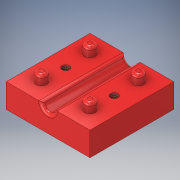
# Autodesk Inventor part: BottomOfSquareSupport
Saved by Autodesk Inventor 2017 SP1 (Build 210196100, 196)
## iProperties
Created: 2015-12-08
Part Number: BottomOfSquareSupport
Material: PC/ABS Plastic
Document SubType Name: Modeling
Designer: steele
Density: 0.357273 g/cm^3
Appearance: Light Red
Author: steele
Autodesk Inventor part; units mm, degrees
ref_plane "YZ Plane" through (0, 0, 0) normal (1, 0, 0) x (0, 1, 0)
ref_plane "XZ Plane" through (0, 0, 0) normal (0, 1, 0) x (-1, 0, 0)
ref_plane "XY Plane" through (0, 0, 0) normal (0, 0, 1) x (1, 0, 0)
sketch "Sketch1" plane through (0, 0, 0) normal (0, 1, 0) x (-1, 0, 0)
  line L0 (-22.225, 22.225) -> (-22.225, -22.225)
  line L1 (-22.225, -22.225) -> (22.225, -22.225)
  line L2 (22.225, -22.225) -> (22.225, 22.225)
  line L3 (22.225, 22.225) -> (-22.225, 22.225)
  line L4 (-22.225, 22.225) -> (22.225, -22.225) construction
  line L5 (-22.225, -22.225) -> (22.225, 22.225) construction
  point P0 (0, 0)
  dimension "d0" = 44.45
  constraints: 12 end point, 2 midpoint, 2 parallel, 2 perpendicular, 1 vertical
  measures "d0" distance of L0.start L0.end
extrude "Extrusion1" add sketch "Sketch1" along normal blind 12.7
sketch "Sketch2" plane through (-22.225, 0, 22.225) normal (0, 0, 1) x (1, 0, 0)
  line L0 (44.45, 12.7) -> (0, 12.7) projected
  arc A0 (18.7325, 12.7) -> (25.7175, 12.7) centre (22.225, 12.7) ccw
  point P0 (22.225, 0)
  dimension "d3" = 6.985
  constraints: 2 point on circle, 2 point on line, 1 centre point, 1 midpoint
  measures "d3" diameter of A0
extrude "Extrusion2" cut sketch "Sketch2" against normal through all
sketch "Sketch3" plane through (0, 0, 0) normal (0, -1, 0) x (1, 0, 0)
  line L0 (-22.225, -22.225) -> (-22.225, 22.225) projected
  line L1 (22.225, 22.225) -> (22.225, -22.225) projected
  line L2 (-22.225, 22.225) -> (-3.4925, 22.225) projected
  line L3 (3.4925, 22.225) -> (22.225, 22.225) projected
  point P0 (0, 0)
  point P1 (-12.8588, 0)
  point P2 (12.8588, 0)
  dimension "d6" = 9.3663
  dimension "d7" = 9.3663
  dimension "d22" = 22.225
  dimension "d23" = 22.225
  measures "d6" distance from line of L0 point (-12.859, 0)
  measures "d7" distance from line of point (12.859, 0) L1
  measures "d22" distance from line of L2 point (-12.859, 0)
  measures "d23" distance from line of L3 point (12.859, 0)
hole "Hole1" at (-12.8588, 0, 0) at (12.8588, 0, 0) direction (0, 1, 0) diameter 3.9624 end through all thread size "10-32 UNF" class "2B" standard "ANSI Unified Screw Threads"
sketch "Sketch7" plane through (0, 12.7, 0) normal (0, 1, 0) x (1, 0, 0)
  line L0 (-12.8588, -12.8588) -> (12.8588, -12.8588) construction
  line L1 (12.8588, -12.8588) -> (12.8588, 12.8588) construction
  line L2 (12.8588, 12.8588) -> (-12.8588, 12.8588) construction
  line L3 (-12.8588, 12.8588) -> (-12.8588, -12.8588) construction
  line L4 (-12.8588, -12.8588) -> (12.8588, 12.8588) construction
  line L5 (12.8588, -12.8588) -> (-12.8588, 12.8588) construction
  line L6 (-22.225, 22.225) -> (-22.225, -22.225) construction
  line L7 (-22.225, -22.225) -> (-3.4925, -22.225) construction
  circle A0 centre (-12.8588, -12.8588) radius 2.7305
  circle A1 centre (-12.8588, 12.8588) radius 2.7305
  circle A2 centre (12.8588, 12.8588) radius 2.7305
  circle A3 centre (12.8588, -12.8588) radius 2.7305
  point P0 (0, 0)
  dimension "d26" = 9.3663
  dimension "d27" = 9.3663
  dimension "d28" = 5.461
  constraints: 12 end point, 4 centre point, 4 coincident, 3 equal radius, 2 midpoint, 2 parallel, 1 horizontal, 1 perpendicular
  measures "d26" distance between parallel lines of L6 L3
  measures "d27" distance between parallel lines of L7 L0
  measures "d28" diameter of A0
extrude "Extrusion3" add sketch "Sketch7" along normal blind 5.08
fillet "Fillet1" radius 1.5875 4 edges at (-15.5892, 17.78, 12.8588) (-15.5892, 17.78, -12.8588) (10.1283, 17.78, -12.8588) (10.1283, 17.78, 12.8588)
fillet "Fillet2" radius 1.5875 4 edges at (-3.4925, 12.7, 0) (3.4925, 12.7, 0) (0, 9.2075, 22.225) (0, 9.2075, -22.225)
sketch "Sketch4" plane through (0, 12.7, 0) normal (0, 1, 0) x (1, 0, 0)
  point P0 (-11.9062, 0)
sketch "Sketch8" plane through (0, 12.7, 0) normal (0, 1, 0) x (1, 0, 0)
  point P0 (13.4937, 0)
equation "\"d0\" = baseWidth"
equation "\"d1\" = heightOfBottomSupport"
equation "\"d3\" = bottomHoleDiam"
equation "\"d4\" = deltaBottomToTop"
equation "\"d6\" = edgeToBoltHole"
equation "\"d7\" = edgeToBoltHole"
equation "\"d22\" = 0.5 * baseWidth"
equation "\"d23\" = 0.5 * baseWidth"
equation "\"d26\" = edgeToBoltHole"
equation "\"d27\" = edgeToBoltHole"
equation "\"d28\" = supportHoleDiam"
equation "\"d29\" = supportHoleLength"
equation "\"bottomHoleDiam\" = 6.985"
equation "\"baseWidth\" = 44.45"
equation "\"height\" = deltaBottomToTop + heightOfBottomHole + heightOfTopHole"
equation "\"deltaBottomToTop\" = 25.4"
equation "\"topHoleDiam\" = 9.525"
equation "\"edgeToBoltHole\" = -0.25 * bottomHoleDiam + 0.25 * baseWidth"
equation "\"washerDiam\" = 13.97"
equation "\"depthForSocketHead\" = 6.35"
equation "\"xbottomHoleDiam\" = 9.525"
equation "\"baseLength\" = 38.1"
equation "\"heightOfBottomSupport\" = 12.7"
equation "\"supportHoleDiam\" = 5.461"
equation "\"supportHoleLength\" = 5.08"
equation "\"heightOfBottomHole\" = 9.8425"
equation "\"heightOfTopHole\" = 9.8425"
body "Solid1"
